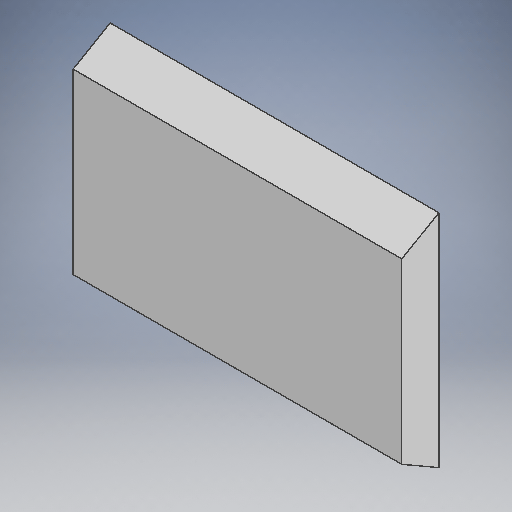
# Autodesk Inventor part: door
Saved by Autodesk Inventor 2025.2 (Build 292293000, 293)
## iProperties
Created: 2025-03-09
Part Number: door
Material: Generic
Document SubType Name: Modeling
Designer: Alex
Density: 1 g/cm^3
Appearance: Default
Author: Alex
Autodesk Inventor part; units mm, degrees
ref_plane "YZ Plane" through (0, 0, 0) normal (1, 0, 0) x (0, 1, 0)
ref_plane "XZ Plane" through (0, 0, 0) normal (0, 1, 0) x (-1, 0, 0)
ref_plane "XY Plane" through (0, 0, 0) normal (0, 0, 1) x (1, 0, 0)
sketch "Sketch1" plane through (0, 0, 0) normal (1, 0, 0) x (0, 1, 0)
  line L0 (0, 0) -> (1.7321, 3) construction
  line L1 (1.7321, 3) -> (15.2679, 3) construction
  line L2 (15.2679, 3) -> (17, 0) construction
  line L3 (17, 0) -> (0, 0) construction
  line L4 (15.2679, 3) -> (15.2679, 0) construction
  line L5 (0.1732, 0.1) -> (1.7898, 2.9)
  line L6 (1.7898, 2.9) -> (15.2102, 2.9)
  line L7 (15.2102, 2.9) -> (16.8268, 0.1)
  line L8 (16.8268, 0.1) -> (0.1732, 0.1)
  dimension "d0" = 60
  dimension "d1" = 17
  dimension "d2" = 3
  dimension "d11" = 0.1
  constraints: 18 end point, 2 parallel, 1 equal length, 1 horizontal, 1 perpendicular, 1 point on line, 3 other
  measures "d0" angle of L3 L0
  measures "d1" distance of L0.start L2.end
  measures "d2" distance of L1.end L4.end
  measures "d11" distance between parallel lines of L3 L8
extrude "Extrusion1" add sketch "Sketch1" along normal blind 24.8
body "Solid1"
